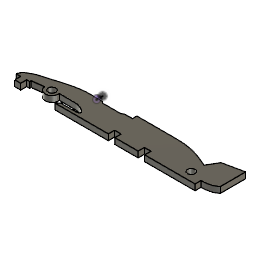
side (Autodesk Fusion 360 design; units mm, degrees)
Autodesk Fusion 360 part; units mm, degrees
sketch "Sketch1" plane through (0, 0, 0) normal (0, 0, 1) x (1, 0, 0)
  line L0 (0, 0) -> (0, 2)
  dimension "d1" = 2
  constraint coincident L0.start origin
  constraint vertical L0
  measures "d1" distance of L0.start L0.end
sketch "Sketch2" plane through (0, 0, 0) normal (0, 0, 1) x (1, 0, 0)
  line L0 (-4, -10) -> (43, -10)
  line L1 (43, -10) -> (43, -8)
  line L2 (47.9756, 2.0171) -> (48, -6.5)
  line L3 (39.0303, -3.0135) -> (24.9995, 2.9996)
  line L4 (24.9995, 2.9996) -> (15, 2.9996)
  line L5 (15, 2.9996) -> (15, 1)
  line L6 (15, 1) -> (16, 1)
  line L7 (16, 1) -> (17, 0)
  line L8 (17, 0) -> (13.5, 0)
  line L9 (13.5, 0) -> (13.5, -1.5)
  line L10 (13.5, -1.5) -> (11, -1.5)
  line L11 (11, -1.5) -> (10, -2)
  line L12 (10, -2) -> (4, -2)
  line L13 (4, -2) -> (3.5, -1.5)
  line L14 (3.5, -1.5) -> (-2, -1.5)
  line L15 (-22, -8) -> (-21.5, -8)
  line L16 (-21.5, -8) -> (-21.5, -9.5)
  line L17 (-21.5, -9.5) -> (-19.5, -9.5)
  line L18 (-19.5, -9.5) -> (-19.5, -8)
  line L19 (-19.5, -8) -> (-17.5, -8)
  line L20 (-17.5, -8) -> (-17.5, -9.5)
  line L21 (-17.5, -9.5) -> (-15.5, -9.5)
  line L22 (-15.5, -9.5) -> (-15.5, -8)
  line L23 (-15.5, -8) -> (-14.5, -8)
  line L24 (-14.5, -8) -> (-14.5, -7.5)
  line L25 (-14.5, -7.5) -> (-10.5, -7)
  spline S0 degree 5 poles (43, -8) (43.1243, -8) (43.3709, -7.9973) (43.7346, -7.9856) (44.2067, -7.9543) (44.7742, -7.8873) (45.3167, -7.7897) (45.8323, -7.6588) (46.3191, -7.4927) (46.778, -7.2921) (47.2108, -7.0593) (47.5377, -6.8494) (47.7727, -6.6795) (47.925, -6.5607) (48, -6.5) knots 0 0 0 0 0 0 0.1 0.2 0.3 0.4 0.5 0.6 0.7 0.8 0.9 1 1 1 1 1 1
  spline S1 degree 5 poles (-2, -1.5) (-2.3206, -1.5261) (-2.956, -1.5878) (-3.8921, -1.7095) (-5.1165, -1.9289) (-6.6646, -2.2931) (-8.2984, -2.739) (-10.0755, -3.2574) (-12.0257, -3.8347) (-14.1206, -4.4614) (-16.2745, -5.11) (-18.3909, -5.7232) (-20.3509, -6.2532) (-22.0238, -6.6774) (-23.2636, -7.0373) (-23.9224, -7.4411) (-23.8411, -8.0289) (-23.5912, -8.3172) (-23.3733, -8.3788) (-23.2517, -8.3768) knots 0 0 0 0 0 0 0.066667 0.133333 0.2 0.266667 0.333333 0.4 0.466667 0.533333 0.6 0.666667 0.733333 0.8 0.866667 0.933333 1 1 1 1 1 1
  line L26 (0.3407, -1.3098) -> (-4.3407, -1.6902)
  line L27 (-22.5, -6.5) -> (-24.5366, -8.0384)
  line L28 (-25.672, -8.4178) -> (-20.8314, -8.3357)
  line L29 (-9.3658, -3.0439) -> (-15.1499, -4.7669)
  line L30 (-23.2517, -8.3768) -> (-22, -8)
  line L31 (-4, -10) -> (-3, -9)
  spline S2 degree 5 poles (2, -9) (2.0745, -9) (2.2233, -8.9958) (2.4466, -8.977) (2.7143, -8.9327) (2.9127, -8.8588) (2.9525, -8.7626) (3.089, -8.5745) (3.198, -8.299) (3.0445, -7.9753) (2.609, -7.6334) (2.0313, -7.2974) (1.3954, -7.0017) (0.7908, -6.7742) (0.2621, -6.6304) (-0.185, -6.5675) (-0.6263, -6.5452) (-1.1247, -6.5382) (-1.7321, -6.5328) (-2.4901, -6.5238) (-3.4309, -6.5123) (-4.3482, -6.5042) (-5.1351, -6.5008) (-5.7043, -6.5) (-6, -6.5) knots 0 0 0 0 0 0 0.05 0.1 0.15 0.2 0.25 0.3 0.35 0.4 0.45 0.5 0.55 0.6 0.65 0.7 0.75 0.8 0.85 0.9 0.95 1 1 1 1 1 1
  line L32 (-3, -9) -> (2, -9)
  line L33 (0.5, -9) -> (3.5, -9)
  line L34 (2.5806, -9.2421) -> (3.2857, -8.3542)
  line L35 (3.6022, -8.7426) -> (2.3978, -7.2574)
  line L36 (-4, -6.5) -> (-8, -6.5)
  line L37 (0.7, -6.7) -> (-0.7, -6.5)
  line L38 (39.0303, -3.0135) -> (41.1508, 0.5664)
  line L39 (47.9756, 2.0171) -> (41.1508, 0.5664)
  line L40 (47.9756, 2.0171) -> (54.9529, 2.0171) construction
  circle A0 centre (-8.25, -6.75) radius 1.25
  circle A1 centre (38.7492, -7.0181) radius 1.25
  arc A2 (-10.4862, -6.9985) -> (-6.0138, -6.5015) centre (-8.25, -6.75) ccw
  line L41 (-10.5, -7) -> (-10.4862, -6.9985)
  line L42 (-6.0138, -6.5015) -> (-6, -6.5)
  point P0 (45.9227, -7.6203)
  point P1 (-12.2579, -3.9054)
  point P2 (-23.5183, -7.2692)
  point P3 (2.9331, -8.7981)
  point P4 (3, -8)
  point P5 (0, -6.6)
  dimension "d4" = 0.5
  dimension "d5" = 168
  dimension "d6" = 4.5
  dimension "d7" = 2.5
  dimension "d8" = 47
  dimension "d9" = 2.5
  constraint horizontal L0
  constraint perpendicular L0 L1
  constraint perpendicular L4 L5
  constraint perpendicular L5 L6
  constraint perpendicular L5 L8
  constraint perpendicular L8 L9
  constraint perpendicular L9 L10
  constraint perpendicular L9 L12
  constraint perpendicular L9 L14
  constraint perpendicular L9 L15
  constraint perpendicular L15 L16
  constraint perpendicular L16 L17
  constraint perpendicular L17 L18
  constraint perpendicular L18 L19
  constraint perpendicular L19 L20
  constraint perpendicular L18 L21
  constraint perpendicular L21 L22
  constraint perpendicular L22 L23
  constraint perpendicular L23 L24
  constraint midpoint L14.end L26
  constraint midpoint P2 L27
  constraint midpoint S1.end L28
  constraint midpoint P1 L29
  constraint parallel L0 L32
  constraint midpoint S2.start L33
  constraint midpoint P3 L34
  constraint midpoint P4 L35
  constraint midpoint S2.end L36
  constraint midpoint P5 L37
  constraint horizontal L40
  constraint concentric A0 A2
  constraint coincident A2.end L41
  constraint collinear L41 L42
  measures "d4" distance of L15.start L15.end
  measures "d5" angle of L39 L40
  measures "d6" diameter of A2
  measures "d7" diameter of A0
  measures "d8" distance of A0.centre A1.centre
  measures "d9" diameter of A1
extrude "Extrude1" add sketch "Sketch2" along normal blind 4 contours L0 L1 L2 L3 L4 L5 L6 L7 L8 L9 L10 L11 L12 L13 L14 L15 L16 L17 L18 L19 L20 L21 L22 L23 L24 L25 S0 S1 L30 L31 S2 L32 L33 L34 L35 L36 L38 L39 A2 L41 L42 | S2 L33 L34 | S2 L34 L35
extrude "Extrude2" cut 3 faces at (18.0352, -6.1228, 4) (2.64, -8.9637, 4) (3.1854, -8.3471, 4) along direction (0, 0, -1) blind 2
sketch "Sketch3" plane through (0, 0, 2) normal (0, 0, 1) x (-1, 0, 0)
  circle A0 centre (8.25, 6.75) radius 1.25
  circle A1 centre (-38.7492, 7.0181) radius 1.25
  line L0 (-39.0303, 3.0135) -> (-24.9995, -2.9996)
  line L1 (-24.9995, -2.9996) -> (-15, -2.9996)
  line L2 (-15, -2.9996) -> (-15, -1)
  line L3 (-15, -1) -> (-16, -1)
  line L4 (-16, -1) -> (-17, 0)
  line L5 (-17, 0) -> (-13.5, 0)
  line L6 (-13.5, 0) -> (-13.5, 1.5)
  line L7 (-13.5, 1.5) -> (-11, 1.5)
  line L8 (-11, 1.5) -> (-10, 2)
  line L9 (-10, 2) -> (-4, 2)
  line L10 (-4, 2) -> (-3.5, 1.5)
  line L11 (-3.5, 1.5) -> (2, 1.5)
  spline S0 degree 3 poles (23.2517, 8.3768) (23.2913, 8.3774) (23.3306, 8.3739) (23.4065, 8.3574) (23.4422, 8.345) (23.538, 8.2981) (23.592, 8.2549) (23.6937, 8.1395) (23.7366, 8.0627) (23.7887, 7.9091) (23.8011, 7.8316) (23.796, 7.683) (23.7807, 7.6134) (23.7174, 7.4694) (23.6664, 7.402) (23.4902, 7.2322) (23.3255, 7.1371) (22.7078, 6.8769) (22.116, 6.7122) (17.749, 5.5568) (15.9897, 5.0181) (6.9369, 2.3188) (4.8851, 1.7345) (2, 1.5) knots -1.822885 -1.822885 -1.822885 -1.822885 -1.805431 -1.805431 -1.788714 -1.788714 -1.758445 -1.758445 -1.720867 -1.720867 -1.686971 -1.686971 -1.655485 -1.655485 -1.618043 -1.618043 -1.548324 -1.548324 -1.421892 -1.421892 -0.868391 -0.868391 0 0 0 0
  line L12 (23.2517, 8.3768) -> (22, 8)
  line L13 (22, 8) -> (21.5, 8)
  line L14 (21.5, 8) -> (21.5, 9.5)
  line L15 (21.5, 9.5) -> (19.5, 9.5)
  line L16 (19.5, 9.5) -> (19.5, 8)
  line L17 (19.5, 8) -> (17.5, 8)
  line L18 (17.5, 8) -> (17.5, 9.5)
  line L19 (17.5, 9.5) -> (15.5, 9.5)
  line L20 (15.5, 9.5) -> (15.5, 8)
  line L21 (15.5, 8) -> (14.5, 8)
  line L22 (14.5, 8) -> (14.5, 7.5)
  line L23 (14.5, 7.5) -> (10.5, 7)
  line L24 (10.5, 7) -> (10.4862, 6.9985)
  arc A2 (10.4862, 6.9985) -> (6.0138, 6.5015) centre (8.25, 6.75) ccw
  line L25 (6.0138, 6.5015) -> (6, 6.5)
  spline S1 degree 3 poles (-2, 9) (-2.307, 9) (-2.6056, 8.9574) (-2.8195, 8.8857) (-2.8535, 8.868) (-2.9146, 8.8251) (-2.9379, 8.7949) (-2.9899, 8.7151) (-3.0528, 8.6192) (-3.1122, 8.4823) (-3.1281, 8.431) (-3.1401, 8.3228) (-3.1354, 8.27) (-3.1021, 8.1535) (-3.0679, 8.0879) (-2.9271, 7.9045) (-2.7636, 7.7479) (-1.9988, 7.2763) (-1.4847, 7.0375) (-0.2064, 6.571) (0.3, 6.5494) (1.2987, 6.5368) (3.3305, 6.5) (6, 6.5) knots -26.792041 -26.792041 -26.792041 -26.792041 -20.718739 -20.718739 -18.719435 -18.719435 -15.732492 -15.732492 -13.815618 -13.815618 -12.725518 -12.725518 -11.621731 -11.621731 -10.278934 -10.278934 -8.046978 -8.046978 -5.445174 -5.445174 -0.800838 -0.800838 0 0 0 0
  line L26 (-2, 9) -> (3, 9)
  line L27 (3, 9) -> (4, 10)
  line L28 (4, 10) -> (-43, 10)
  line L29 (-43, 10) -> (-43, 8)
  spline S2 degree 3 poles (-48, 6.5) (-47.1315, 7.2033) (-46.3055, 7.5076) (-44.9417, 7.912) (-43.9649, 7.9996) (-43, 8) knots -0.446877 -0.446877 -0.446877 -0.446877 -0.289476 -0.289476 0 0 0 0
  line L30 (-48, 6.5) -> (-47.9756, -2.0171)
  line L31 (-47.9756, -2.0171) -> (-41.1508, -0.5664)
  line L32 (-41.1508, -0.5664) -> (-39.0303, 3.0135)
  spline S3 degree 5 poles (15.3694, 4.8357) (15.4789, 4.8701) (15.6954, 4.9409) (16.0123, 5.0532) (16.4193, 5.215) (16.9007, 5.4377) (17.3515, 5.6804) (17.7666, 5.9416) (18.1383, 6.2177) (18.4555, 6.5029) (18.7042, 6.7877) (18.8686, 7.061) (18.934, 7.3118) (18.888, 7.5307) (18.7243, 7.7115) (18.4419, 7.8518) (18.1224, 7.9313) (17.8311, 7.9727) (17.6142, 7.9922) (17.5, 8) knots 0 0 0 0 0 0 0.066667 0.133333 0.2 0.266667 0.333333 0.4 0.466667 0.533333 0.6 0.666667 0.733333 0.8 0.866667 0.933333 1 1 1 1 1 1
  point P0 (18.1, 6.2)
  point P1 (18.9, 7.4)
  constraint coincident S0 S3.start
  constraint coincident L17.end L18.start
extrude "Extrude3" cut sketch "Sketch3" against normal blind 2 contours S0 L12 L13 L14 L15 L16 L17 S3
sketch "Sketch4" plane through (0, 0, 2) normal (0, 0, 1) x (-1, 0, 0)
  spline S0 degree 5 poles (15.3694, 4.8357) (15.4789, 4.8701) (15.6954, 4.9409) (16.0123, 5.0532) (16.4193, 5.215) (16.9007, 5.4377) (17.3515, 5.6804) (17.7666, 5.9416) (18.1383, 6.2177) (18.4555, 6.5029) (18.7042, 6.7877) (18.8686, 7.061) (18.934, 7.3118) (18.888, 7.5307) (18.7243, 7.7115) (18.4419, 7.8518) (18.1224, 7.9313) (17.8311, 7.9727) (17.6142, 7.9922) (17.5, 8) knots 0 0 0 0 0 0 0.066667 0.133333 0.2 0.266667 0.333333 0.4 0.466667 0.533333 0.6 0.666667 0.733333 0.8 0.866667 0.933333 1 1 1 1 1 1
  line L0 (17.5, 8) -> (17.5, 9.5)
  line L1 (17.5, 9.5) -> (15.5, 9.5)
  line L2 (15.5, 9.5) -> (15.5, 8)
  line L3 (15.5, 8) -> (14.5, 8)
  line L4 (14.5, 8) -> (14.5, 7.5)
  line L5 (14.5, 7.5) -> (10.5, 7)
  line L6 (10.5, 7) -> (10.4862, 6.9985)
  arc A0 (10.4862, 6.9985) -> (6.0138, 6.5015) centre (8.25, 6.75) ccw
  line L7 (6.0138, 6.5015) -> (6, 6.5)
  spline S1 degree 3 poles (-2, 9) (-2.307, 9) (-2.6056, 8.9574) (-2.8195, 8.8857) (-2.8535, 8.868) (-2.9146, 8.8251) (-2.9379, 8.7949) (-2.9899, 8.7151) (-3.0528, 8.6192) (-3.1122, 8.4823) (-3.1281, 8.431) (-3.1401, 8.3228) (-3.1354, 8.27) (-3.1021, 8.1535) (-3.0679, 8.0879) (-2.9271, 7.9045) (-2.7636, 7.7479) (-1.9988, 7.2763) (-1.4847, 7.0375) (-0.2064, 6.571) (0.3, 6.5494) (1.2987, 6.5368) (3.3305, 6.5) (6, 6.5) knots -26.792041 -26.792041 -26.792041 -26.792041 -20.718739 -20.718739 -18.719435 -18.719435 -15.732492 -15.732492 -13.815618 -13.815618 -12.725518 -12.725518 -11.621731 -11.621731 -10.278934 -10.278934 -8.046978 -8.046978 -5.445174 -5.445174 -0.800838 -0.800838 0 0 0 0
  line L8 (-2, 9) -> (3, 9)
  line L9 (3, 9) -> (4, 10)
  line L10 (4, 10) -> (-43, 10)
  line L11 (-43, 10) -> (-43, 8)
  spline S2 degree 3 poles (-48, 6.5) (-47.1315, 7.2033) (-46.3055, 7.5076) (-44.9417, 7.912) (-43.9649, 7.9996) (-43, 8) knots -0.446877 -0.446877 -0.446877 -0.446877 -0.289476 -0.289476 0 0 0 0
  line L12 (-48, 6.5) -> (-47.9756, -2.0171)
  line L13 (-47.9756, -2.0171) -> (-41.1508, -0.5664)
  line L14 (-41.1508, -0.5664) -> (-39.0303, 3.0135)
  line L15 (-39.0303, 3.0135) -> (-24.9995, -2.9996)
  line L16 (-24.9995, -2.9996) -> (-15, -2.9996)
  line L17 (-15, -2.9996) -> (-15, -1)
  line L18 (-15, -1) -> (-16, -1)
  line L19 (-16, -1) -> (-17, 0)
  line L20 (-17, 0) -> (-13.5, 0)
  line L21 (-13.5, 0) -> (-13.5, 1.5)
  line L22 (-13.5, 1.5) -> (-11, 1.5)
  line L23 (-11, 1.5) -> (-10, 2)
  line L24 (-10, 2) -> (-4, 2)
  line L25 (-4, 2) -> (-3.5, 1.5)
  line L26 (-3.5, 1.5) -> (2, 1.5)
  spline S3 degree 3 poles (15.3694, 4.8357) (14.5023, 4.576) (13.5708, 4.2968) (6.9369, 2.3188) (4.8851, 1.7345) (2, 1.5) knots -1.041963 -1.041963 -1.041963 -1.041963 -0.868391 -0.868391 0 0 0 0
  circle A1 centre (8.25, 6.75) radius 1.25
  circle A2 centre (-38.7492, 7.0181) radius 1.25
  line L27 (-17, 0) -> (-34, 0)
  constraint coincident L19.end L20.start
  constraint parallel L20 L27
extrude "Extrude4" cut sketch "Sketch4" against normal blind 4 contours L15 L16 L17 L18 L19 L27
sketch "Sketch5" plane through (0, 0, 2) normal (0, 0, 1) x (-1, 0, 0)
  line L0 (-31.9987, 0) -> (-13.5, 0)
  line L1 (-13.5, 0) -> (-13.5, 1.5)
  line L2 (-13.5, 1.5) -> (-11, 1.5)
  line L3 (-11, 1.5) -> (-10, 2)
  line L4 (-10, 2) -> (-4, 2)
  line L5 (-4, 2) -> (-3.5, 1.5)
  line L6 (-3.5, 1.5) -> (2, 1.5)
  spline S0 degree 3 poles (15.3694, 4.8357) (14.5023, 4.576) (13.5708, 4.2968) (6.9369, 2.3188) (4.8851, 1.7345) (2, 1.5) knots -1.041963 -1.041963 -1.041963 -1.041963 -0.868391 -0.868391 0 0 0 0
  spline S1 degree 5 poles (15.3694, 4.8357) (15.4789, 4.8701) (15.6954, 4.9409) (16.0123, 5.0532) (16.4193, 5.215) (16.9007, 5.4377) (17.3515, 5.6804) (17.7666, 5.9416) (18.1383, 6.2177) (18.4555, 6.5029) (18.7042, 6.7877) (18.8686, 7.061) (18.934, 7.3118) (18.888, 7.5307) (18.7243, 7.7115) (18.4419, 7.8518) (18.1224, 7.9313) (17.8311, 7.9727) (17.6142, 7.9922) (17.5, 8) knots 0 0 0 0 0 0 0.066667 0.133333 0.2 0.266667 0.333333 0.4 0.466667 0.533333 0.6 0.666667 0.733333 0.8 0.866667 0.933333 1 1 1 1 1 1
  line L7 (17.5, 8) -> (17.5, 9.5)
  line L8 (17.5, 9.5) -> (15.5, 9.5)
  line L9 (15.5, 9.5) -> (15.5, 8)
  line L10 (15.5, 8) -> (14.5, 8)
  line L11 (14.5, 8) -> (14.5, 7.5)
  line L12 (14.5, 7.5) -> (10.5, 7)
  line L13 (10.5, 7) -> (10.4862, 6.9985)
  arc A0 (10.4862, 6.9985) -> (6.0138, 6.5015) centre (8.25, 6.75) ccw
  line L14 (6.0138, 6.5015) -> (6, 6.5)
  spline S2 degree 3 poles (-2, 9) (-2.307, 9) (-2.6056, 8.9574) (-2.8195, 8.8857) (-2.8535, 8.868) (-2.9146, 8.8251) (-2.9379, 8.7949) (-2.9899, 8.7151) (-3.0528, 8.6192) (-3.1122, 8.4823) (-3.1281, 8.431) (-3.1401, 8.3228) (-3.1354, 8.27) (-3.1021, 8.1535) (-3.0679, 8.0879) (-2.9271, 7.9045) (-2.7636, 7.7479) (-1.9988, 7.2763) (-1.4847, 7.0375) (-0.2064, 6.571) (0.3, 6.5494) (1.2987, 6.5368) (3.3305, 6.5) (6, 6.5) knots -26.792041 -26.792041 -26.792041 -26.792041 -20.718739 -20.718739 -18.719435 -18.719435 -15.732492 -15.732492 -13.815618 -13.815618 -12.725518 -12.725518 -11.621731 -11.621731 -10.278934 -10.278934 -8.046978 -8.046978 -5.445174 -5.445174 -0.800838 -0.800838 0 0 0 0
  line L15 (-2, 9) -> (3, 9)
  line L16 (3, 9) -> (4, 10)
  line L17 (4, 10) -> (-43, 10)
  line L18 (-43, 10) -> (-43, 8)
  spline S3 degree 3 poles (-48, 6.5) (-47.1315, 7.2033) (-46.3055, 7.5076) (-44.9417, 7.912) (-43.9649, 7.9996) (-43, 8) knots -0.446877 -0.446877 -0.446877 -0.446877 -0.289476 -0.289476 0 0 0 0
  line L19 (-48, 6.5) -> (-47.9756, -2.0171)
  line L20 (-47.9756, -2.0171) -> (-41.1508, -0.5664)
  line L21 (-41.1508, -0.5664) -> (-39.0303, 3.0135)
  line L22 (-39.0303, 3.0135) -> (-31.9987, 0)
  circle A1 centre (8.25, 6.75) radius 1.25
  circle A2 centre (-38.7492, 7.0181) radius 1.25
  line L23 (0, 0) -> (-15, 0)
  line L24 (-15, 0) -> (-15, 10)
  line L25 (-15, 10) -> (0, 10)
  line L26 (0, 10) -> (0, 0)
  line L27 (0, 0) -> (-25, 0)
  line L28 (-25, 0) -> (-25, 10)
  line L29 (-25, 10) -> (0, 10)
  line L30 (0, 10) -> (0, 0)
  line L31 (-14, 8) -> (-16, 8)
  line L32 (-16, 8) -> (-16, 10)
  line L33 (-16, 10) -> (-14, 10)
  line L34 (-14, 10) -> (-14, 8)
  line L35 (-24, 8) -> (-26, 8)
  line L36 (-26, 8) -> (-26, 10)
  line L37 (-26, 10) -> (-24, 10)
  line L38 (-24, 10) -> (-24, 8)
  line L39 (-16.1, 10.1) -> (-13.9, 10.1)
  line L40 (-13.9, 10.1) -> (-13.9, 7.9)
  line L41 (-13.9, 7.9) -> (-16.1, 7.9)
  line L42 (-16.1, 7.9) -> (-16.1, 10.1)
  line L43 (-26.1, 10.1) -> (-23.9, 10.1)
  line L44 (-23.9, 10.1) -> (-23.9, 7.9)
  line L45 (-23.9, 7.9) -> (-26.1, 7.9)
  line L46 (-26.1, 7.9) -> (-26.1, 10.1)
  dimension "d18" = 15
  dimension "d19" = 10
  dimension "d20" = 25
  dimension "d21" = 10
  dimension "d22" = -0.1
  dimension "d23" = -0.1
  constraint horizontal L23
  constraint vertical L24
  constraint horizontal L25
  constraint vertical L26
  constraint coincident L23.start L26.end
  constraint horizontal L27
  constraint vertical L28
  constraint horizontal L29
  constraint vertical L30
  constraint horizontal L31
  constraint vertical L32
  constraint horizontal L33
  constraint vertical L34
  constraint horizontal L35
  constraint vertical L36
  constraint horizontal L37
  constraint vertical L38
  constraint coincident L17 L36.end
  measures "d18" distance of L23.start L23.end
  measures "d19" distance of L23.start L25.end
  measures "d20" distance of L23.start L27.end
  measures "d21" distance of L23.start L25.end
extrude "Extrude5" cut sketch "Sketch5" against normal blind 2 contours L17 L28 L35 L36 L45 L46 | L17 L28 L29 L35 L38 L44 L45 | L17 L24 L29 L31 L32 L41 L42 | L17 L24 L25 L29 L31 L34 L40 L41 | L17 L28 L35 L36 L37 | L17 L28 L29 L35 L37 L38 | L17 L24 L29 L31 L32 L33 | L17 L24 L25 L29 L31 L33 L34
fillet "Fillet1" radius 24.25 1 edges at (31.9987, 0, 1)
extrude "Extrude6" add 1 faces at (-16.8333, -9.5, 0.6667) along direction (0, -1, 0) blind 0.5
sketch "Sketch6" plane through (0, 0, 2) normal (0, 0, 1) x (-1, 0, 0)
  arc A0 (-36.5737, 1.9607) -> (-27.0212, 0) centre (-27.0212, 24.25) ccw
  line L0 (-27.0212, 0) -> (-13.5, 0)
  line L1 (-13.5, 0) -> (-13.5, 1.5)
  line L2 (-13.5, 1.5) -> (-11, 1.5)
  line L3 (-11, 1.5) -> (-10, 2)
  line L4 (-10, 2) -> (-4, 2)
  line L5 (-4, 2) -> (-3.5, 1.5)
  line L6 (-3.5, 1.5) -> (2, 1.5)
  spline S0 degree 3 poles (15.3694, 4.8357) (14.5023, 4.576) (13.5708, 4.2968) (6.9369, 2.3188) (4.8851, 1.7345) (2, 1.5) knots -1.041963 -1.041963 -1.041963 -1.041963 -0.868391 -0.868391 0 0 0 0
  spline S1 degree 5 poles (15.3694, 4.8357) (15.4789, 4.8701) (15.6954, 4.9409) (16.0123, 5.0532) (16.4193, 5.215) (16.9007, 5.4377) (17.3515, 5.6804) (17.7666, 5.9416) (18.1383, 6.2177) (18.4555, 6.5029) (18.7042, 6.7877) (18.8686, 7.061) (18.934, 7.3118) (18.888, 7.5307) (18.7243, 7.7115) (18.4419, 7.8518) (18.1224, 7.9313) (17.8311, 7.9727) (17.6142, 7.9922) (17.5, 8) knots 0 0 0 0 0 0 0.066667 0.133333 0.2 0.266667 0.333333 0.4 0.466667 0.533333 0.6 0.666667 0.733333 0.8 0.866667 0.933333 1 1 1 1 1 1
  line L7 (17.5, 8) -> (17.5, 10)
  line L8 (17.5, 10) -> (15.5, 10)
  line L9 (15.5, 10) -> (15.5, 8)
  line L10 (15.5, 8) -> (14.5, 8)
  line L11 (14.5, 8) -> (14.5, 7.5)
  line L12 (14.5, 7.5) -> (10.5, 7)
  line L13 (10.5, 7) -> (10.4862, 6.9985)
  arc A1 (10.4862, 6.9985) -> (6.0138, 6.5015) centre (8.25, 6.75) ccw
  line L14 (6.0138, 6.5015) -> (6, 6.5)
  spline S2 degree 3 poles (-2, 9) (-2.307, 9) (-2.6056, 8.9574) (-2.8195, 8.8857) (-2.8535, 8.868) (-2.9146, 8.8251) (-2.9379, 8.7949) (-2.9899, 8.7151) (-3.0528, 8.6192) (-3.1122, 8.4823) (-3.1281, 8.431) (-3.1401, 8.3228) (-3.1354, 8.27) (-3.1021, 8.1535) (-3.0679, 8.0879) (-2.9271, 7.9045) (-2.7636, 7.7479) (-1.9988, 7.2763) (-1.4847, 7.0375) (-0.2064, 6.571) (0.3, 6.5494) (1.2987, 6.5368) (3.3305, 6.5) (6, 6.5) knots -26.792041 -26.792041 -26.792041 -26.792041 -20.718739 -20.718739 -18.719435 -18.719435 -15.732492 -15.732492 -13.815618 -13.815618 -12.725518 -12.725518 -11.621731 -11.621731 -10.278934 -10.278934 -8.046978 -8.046978 -5.445174 -5.445174 -0.800838 -0.800838 0 0 0 0
  line L15 (-2, 9) -> (3, 9)
  line L16 (3, 9) -> (4, 10)
  line L17 (4, 10) -> (-13.9, 10)
  line L18 (-13.9, 10) -> (-13.9, 7.9)
  line L19 (-13.9, 7.9) -> (-16.1, 7.9)
  line L20 (-16.1, 7.9) -> (-16.1, 10)
  line L21 (-16.1, 10) -> (-23.9, 10)
  line L22 (-23.9, 10) -> (-23.9, 7.9)
  line L23 (-23.9, 7.9) -> (-26.1, 7.9)
  line L24 (-26.1, 7.9) -> (-26.1, 10)
  line L25 (-26.1, 10) -> (-43, 10)
  line L26 (-43, 10) -> (-43, 8)
  spline S3 degree 3 poles (-48, 6.5) (-47.1315, 7.2033) (-46.3055, 7.5076) (-44.9417, 7.912) (-43.9649, 7.9996) (-43, 8) knots -0.446877 -0.446877 -0.446877 -0.446877 -0.289476 -0.289476 0 0 0 0
  line L27 (-48, 6.5) -> (-47.9756, -2.0171)
  line L28 (-47.9756, -2.0171) -> (-41.1508, -0.5664)
  line L29 (-41.1508, -0.5664) -> (-39.0303, 3.0135)
  line L30 (-39.0303, 3.0135) -> (-36.5737, 1.9607)
  circle A2 centre (8.25, 6.75) radius 1.25
  circle A3 centre (-38.7492, 7.0181) radius 1.25
  line L31 (14.5, 8) -> (19.5, 8)
  spline S4 degree 5 poles (19, 8) (18.9913, 7.9294) (18.9681, 7.789) (18.9161, 7.5804) (18.8119, 7.3067) (18.6199, 6.9724) (18.3614, 6.6463) (18.0328, 6.329) (17.6349, 6.0203) (17.173, 5.7197) (16.653, 5.4263) (16.1949, 5.1968) (15.8292, 5.0275) (15.5758, 4.9158) (15.4467, 4.8603) knots 0 0 0 0 0 0 0.1 0.2 0.3 0.4 0.5 0.6 0.7 0.8 0.9 1 1 1 1 1 1
  point P0 (18.2, 6.5)
  constraint coincident L10.end L11.start
  constraint perpendicular L7 L31
  constraint coincident L31 S4.start
  constraint coincident S1 S4.end
extrude "Extrude7" add sketch "Sketch6" against normal blind 2 contours S1 L31 S4
extrude "Extrude8" cut sketch "Sketch6" against normal blind 2 contours S1 S4
